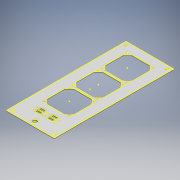
# Autodesk Inventor part: top_panel2
Saved by Autodesk Inventor 2018 (Build 220112000, 112)
## iProperties
Created: 2021-05-16
Part Number: top_panel2
Material: Generic
Document SubType Name: Modeling
Designer: gisen
Density: 1 g/cm^3
Appearance: Default
Author: gisen
Autodesk Inventor part; units mm, degrees
ref_plane "YZ Plane" through (0, 0, 0) normal (1, 0, 0) x (0, 1, 0)
ref_plane "XZ Plane" through (0, 0, 0) normal (0, 1, 0) x (-1, 0, 0)
ref_plane "XY Plane" through (0, 0, 0) normal (0, 0, 1) x (1, 0, 0)
sketch "Sketch1" plane through (0, 0, 0) normal (0, 0, 1) x (1, 0, 0)
  line L0 (-78, 195) -> (78, 195)
  line L1 (78, 195) -> (78, -195)
  line L2 (78, -195) -> (-78, -195)
  line L3 (-78, -195) -> (-78, 195)
  line L4 (-78, 195) -> (78, -195) construction
  line L5 (78, 195) -> (-78, -195) construction
  point P0 (0, 0)
  dimension "d1" = 156
  dimension "d2" = 390
  constraints: 12 end point, 2 midpoint, 2 parallel, 1 horizontal, 1 perpendicular
  measures "d1" distance of L0.start L0.end
  measures "d2" distance of L0.end L1.end
extrude "Extrusion1" add sketch "Sketch1" along normal blind 3
sketch "Sketch2" plane through (0, 0, 3) normal (0, 0, 1) x (1, 0, 0)
  line L0 (-78, -195) -> (78, -195) projected
  line L1 (-78, 195) -> (-78, -195) projected
  arc A0 (-64.4298, -185.2577) -> (-68.2577, -181.4298) centre (-66, -183) ccw
  arc A1 (-69.8472, -183.7153) -> (-66.7153, -186.8472) centre (-68, -185) ccw
  line L2 (-66.7153, -186.8472) -> (-64.4298, -185.2577)
  line L3 (-69.8472, -183.7153) -> (-68.2577, -181.4298)
  line L4 (0, 16.0888) -> (0, -25.3045)
  line L5 (-19.6832, 0) -> (22.709, 0)
  arc A2 (68.2577, -181.4298) -> (64.4298, -185.2577) centre (66, -183) ccw
  arc A3 (66.7153, -186.8472) -> (69.8472, -183.7153) centre (68, -185) ccw
  line L6 (66.7153, -186.8472) -> (64.4298, -185.2577)
  line L7 (69.8472, -183.7153) -> (68.2577, -181.4298)
  arc A4 (-68.2577, 181.4298) -> (-64.4298, 185.2577) centre (-66, 183) ccw
  arc A5 (-66.7153, 186.8472) -> (-69.8472, 183.7153) centre (-68, 185) ccw
  line L8 (-66.7153, 186.8472) -> (-64.4298, 185.2577)
  line L9 (-69.8472, 183.7153) -> (-68.2577, 181.4298)
  arc A6 (64.4298, 185.2577) -> (68.2577, 181.4298) centre (66, 183) ccw
  arc A7 (69.8472, 183.7153) -> (66.7153, 186.8472) centre (68, 185) ccw
  line L10 (66.7153, 186.8472) -> (64.4298, 185.2577)
  line L11 (69.8472, 183.7153) -> (68.2577, 181.4298)
  point P0 (0, 0)
  dimension "d11" = 12
  dimension "d12" = 10
  dimension "d13" = 12
  dimension "d14" = 10
  dimension "d15" = 5.5
  dimension "d16" = 4.5
  constraints: 24 symmetric about line, 20 end point, 16 point on circle, 8 centre point, 8 coincident, 4 tangent, 1 horizontal, 1 vertical, 6 other
  measures "d11" distance from line of L0 point (-66, -183)
  measures "d12" distance from line of L0 point (-68, -185)
  measures "d13" distance from line of L1 point (-66, -183)
  measures "d14" distance from line of L1 point (-68, -185)
  measures "d15" diameter of A0
  measures "d16" diameter of A1
extrude "Extrusion2" cut sketch "Sketch2" against normal up to surface (3 mm away)
sketch "Sketch3" plane through (0, 0, 3) normal (0, 0, 1) x (1, 0, 0)
  line L0 (78, 195) -> (-78, 195) projected
  line L1 (28.4765, 166.7) -> (-28.4765, 166.7)
  circle A0 centre (-41.25, 163.25) radius 2.25
  line L2 (-28.4765, 77.3) -> (28.4765, 77.3)
  circle A1 centre (-41.25, 80.75) radius 2.25
  circle A2 centre (41.25, 80.75) radius 2.25
  circle A3 centre (41.25, 163.25) radius 2.25
  line L3 (44.7, 93.5235) -> (44.7, 150.4765)
  line L4 (-44.7, 150.4765) -> (-44.7, 93.5235)
  arc A4 (28.4765, 77.3) -> (44.7, 93.5235) centre (0, 122) ccw
  arc A5 (44.7, 150.4765) -> (28.4765, 166.7) centre (0, 122) ccw
  arc A6 (-28.4765, 166.7) -> (-44.7, 150.4765) centre (0, 122) ccw
  arc A7 (-44.7, 93.5235) -> (-28.4765, 77.3) centre (0, 122) ccw
  line L5 (28.4765, -17.7) -> (-28.4765, -17.7)
  circle A8 centre (-41.25, -14.25) radius 2.25
  line L6 (-28.4765, 71.7) -> (28.4765, 71.7)
  circle A9 centre (-41.25, 68.25) radius 2.25
  circle A10 centre (41.25, 68.25) radius 2.25
  circle A11 centre (41.25, -14.25) radius 2.25
  line L7 (44.7, 55.4765) -> (44.7, -1.4765)
  line L8 (-44.7, -1.4765) -> (-44.7, 55.4765)
  arc A12 (44.7, 55.4765) -> (28.4765, 71.7) centre (0, 27) ccw
  arc A13 (28.4765, -17.7) -> (44.7, -1.4765) centre (0, 27) ccw
  arc A14 (-44.7, -1.4765) -> (-28.4765, -17.7) centre (0, 27) ccw
  arc A15 (-28.4765, 71.7) -> (-44.7, 55.4765) centre (0, 27) ccw
  circle A16 centre (41.25, -109.25) radius 2.25
  arc A17 (28.4765, -112.7) -> (44.7, -96.4765) centre (0, -68) ccw
  line L9 (44.7, -96.4765) -> (44.7, -39.5235)
  line L10 (-28.4765, -112.7) -> (28.4765, -112.7)
  circle A18 centre (41.25, -26.75) radius 2.25
  arc A19 (44.7, -39.5235) -> (28.4765, -23.3) centre (0, -68) ccw
  circle A20 centre (-41.25, -109.25) radius 2.25
  arc A21 (-44.7, -96.4765) -> (-28.4765, -112.7) centre (0, -68) ccw
  line L11 (-44.7, -39.5235) -> (-44.7, -96.4765)
  line L12 (28.4765, -23.3) -> (-28.4765, -23.3)
  circle A22 centre (-41.25, -26.75) radius 2.25
  arc A23 (-28.4765, -23.3) -> (-44.7, -39.5235) centre (0, -68) ccw
  point P0 (0, 0)
  dimension "d20" = 73
  dimension "d21" = 41.25
  dimension "d22" = 41.25
  dimension "d24" = 44.7
  dimension "d25" = 4.5
  dimension "d27" = 44.7
  dimension "d31" = 360
  constraints: 24 centre point, 24 end point, 24 point on circle, 13 coincident, 2 horizontal, 1 perpendicular, 1 vertical, 13 other
  measures "d20" distance from line of point (0, 122) L0
  measures "d21" horizontal distance of point (0, 122) point (-41.25, 163.25)
  measures "d22" horizontal distance of point (0, 122) point (-41.25, 163.25)
  measures "d24" distance from line of point (0, 122) L1
  measures "d25" diameter of A0
  measures "d27" distance from line of point (0, 122) L2
extrude "Extrusion3" cut sketch "Sketch3" against normal up to surface (3 mm away)
sketch "Sketch4" plane through (0, 0, 3) normal (0, 0, 1) x (1, 0, 0)
  line L0 (-28.5, -131.3505) -> (-11.5, -131.3505)
  line L1 (-11.5, -131.3505) -> (-11.5, -140.3505)
  line L2 (-11.5, -140.3505) -> (-28.5, -140.3505)
  line L3 (-28.5, -140.3505) -> (-28.5, -131.3505)
  line L4 (-28.5, -131.3505) -> (-11.5, -140.3505) construction
  line L5 (-11.5, -131.3505) -> (-28.5, -140.3505) construction
  circle A0 centre (-35, -135.8505) radius 1.65
  circle A1 centre (-5, -135.8505) radius 1.65
  line L6 (0, -126.9429) -> (0, -150.2324)
  line L7 (28.5, -131.3505) -> (11.5, -131.3505)
  line L8 (11.5, -131.3505) -> (11.5, -140.3505)
  line L9 (11.5, -140.3505) -> (28.5, -140.3505)
  line L10 (28.5, -140.3505) -> (28.5, -131.3505)
  line L11 (28.5, -131.3505) -> (11.5, -140.3505) construction
  line L12 (11.5, -131.3505) -> (28.5, -140.3505) construction
  circle A2 centre (35, -135.8505) radius 1.65
  circle A3 centre (5, -135.8505) radius 1.65
  line L13 (-30.7879, -141.8505) -> (-3.35, -141.8505)
  line L14 (-28.5, -152.3505) -> (-11.5, -152.3505)
  line L15 (-11.5, -152.3505) -> (-11.5, -143.3505)
  line L16 (-11.5, -143.3505) -> (-28.5, -143.3505)
  line L17 (-28.5, -143.3505) -> (-28.5, -152.3505)
  line L18 (-28.5, -152.3505) -> (-11.5, -143.3505) construction
  line L19 (-11.5, -152.3505) -> (-28.5, -143.3505) construction
  circle A4 centre (-35, -147.8505) radius 1.65
  circle A5 centre (-5, -147.8505) radius 1.65
  line L20 (28.5, -152.3505) -> (11.5, -152.3505)
  line L21 (11.5, -152.3505) -> (11.5, -143.3505)
  line L22 (11.5, -143.3505) -> (28.5, -143.3505)
  line L23 (28.5, -143.3505) -> (28.5, -152.3505)
  line L24 (28.5, -152.3505) -> (11.5, -143.3505) construction
  line L25 (11.5, -152.3505) -> (28.5, -143.3505) construction
  circle A6 centre (35, -147.8505) radius 1.65
  circle A7 centre (5, -147.8505) radius 1.65
  point P0 (0, 0)
  point P1 (-20, -135.8505)
  point P2 (20, -135.8505)
  point P3 (-20, -147.8505)
  point P4 (20, -147.8505)
  dimension "d37" = 17
  dimension "d38" = 9
  dimension "d39" = 6.5
  dimension "d40" = 4.5
  dimension "d41" = 3.3
  dimension "d42" = 6.5
  dimension "d43" = 4.5
  dimension "d44" = 3.3
  dimension "d45" = 5
  dimension "d46" = 1.5
  constraints: 52 end point, 27 symmetric about line, 8 centre point, 8 coincident, 8 midpoint, 2 horizontal, 2 parallel, 1 perpendicular, 1 vertical, 6 other
  measures "d37" distance of L1.end L2.end
  measures "d38" distance of L0.end L1.end
  measures "d39" distance from line of L3 point (-35, -135.851)
  measures "d40" distance from line of point (-35, -135.851) L0
  measures "d41" diameter of A0
  measures "d42" distance from line of point (-5, -135.851) L1
  measures "d43" distance from line of L0 point (-5, -135.851)
  measures "d44" diameter of A1
  measures "d45" horizontal distance of A1.centre point (0, 0)
  measures "d46" distance between parallel lines of L13 L2
extrude "Extrusion4" cut sketch "Sketch4" against normal up to surface (3 mm away)
sketch "Sketch5" plane through (0, 0, 3) normal (0, 0, 1) x (1, 0, 0)
  line L0 (-78, -195) -> (78, -195) projected
  line L1 (-2.4755, -172.54) -> (2.4755, -172.54)
  line L2 (-2.4755, -187.46) -> (2.4755, -187.46)
  arc A0 (-2.4755, -172.54) -> (-2.4755, -187.46) centre (0, -180) ccw
  arc A1 (2.4755, -187.46) -> (2.4755, -172.54) centre (0, -180) ccw
  point P0 (0, 0)
  dimension "d49" = 15
  dimension "d51" = 7.46
  dimension "d52" = 7.46
  constraints: 4 end point, 4 point on circle, 2 centre point, 2 horizontal, 1 coincident
  measures "d49" distance from line of L0 point (0, -180)
  measures "d51" distance from line of A0.centre L1
  measures "d52" distance from line of point (0, -180) L2
extrude "Extrusion5" cut sketch "Sketch5" against normal up to surface (3 mm away)
sketch "Sketch6" plane through (0, 0, 3) normal (0, 0, 1) x (1, 0, 0)
  line L0 (-2.4755, -172.54) -> (2.4755, -172.54) projected
  arc A0 (2.4755, -187.46) -> (2.4755, -172.54) centre (0, -180) ccw projected
  line L1 (2.4755, -187.46) -> (-2.4755, -187.46) projected
  arc A1 (-2.4755, -172.54) -> (-2.4755, -187.46) centre (0, -180) ccw projected
  line L2 (-11.5, -152.3505) -> (-28.5, -152.3505) projected
  line L3 (-28.5, -152.3505) -> (-28.5, -143.3505) projected
  line L4 (-28.5, -143.3505) -> (-11.5, -143.3505) projected
  line L5 (-11.5, -143.3505) -> (-11.5, -152.3505) projected
  line L6 (11.5, -143.3505) -> (28.5, -143.3505) projected
  line L7 (28.5, -143.3505) -> (28.5, -152.3505) projected
  line L8 (28.5, -152.3505) -> (11.5, -152.3505) projected
  line L9 (11.5, -152.3505) -> (11.5, -143.3505) projected
  line L10 (11.5, -131.3505) -> (28.5, -131.3505) projected
  line L11 (28.5, -131.3505) -> (28.5, -140.3505) projected
  line L12 (28.5, -140.3505) -> (11.5, -140.3505) projected
  line L13 (11.5, -140.3505) -> (11.5, -131.3505) projected
  circle A2 centre (35, -147.8505) radius 1.65 projected
  circle A3 centre (-35, -147.8505) radius 1.65 projected
  circle A4 centre (5, -135.8505) radius 1.65 projected
  circle A5 centre (-5, -135.8505) radius 1.65 projected
  circle A6 centre (-35, -135.8505) radius 1.65 projected
  circle A7 centre (35, -135.8505) radius 1.65 projected
  circle A8 centre (-5, -147.8505) radius 1.65 projected
  circle A9 centre (5, -147.8505) radius 1.65 projected
  line L14 (-11.5, -131.3505) -> (-11.5, -140.3505) projected
  line L15 (-11.5, -140.3505) -> (-28.5, -140.3505) projected
  line L16 (-28.5, -140.3505) -> (-28.5, -131.3505) projected
  line L17 (-28.5, -131.3505) -> (-11.5, -131.3505) projected
  line L18 (28.4765, -17.7) -> (-28.4765, -17.7) projected
  arc A10 (-44.7, -1.4765) -> (-28.4765, -17.7) centre (0, 27) ccw projected
  line L19 (-44.7, -1.4765) -> (-44.7, 55.4765) projected
  arc A11 (-28.4765, 71.7) -> (-44.7, 55.4765) centre (0, 27) ccw projected
  line L20 (-28.4765, 71.7) -> (28.4765, 71.7) projected
  arc A12 (44.7, 55.4765) -> (28.4765, 71.7) centre (0, 27) ccw projected
  line L21 (44.7, 55.4765) -> (44.7, -1.4765) projected
  arc A13 (28.4765, -17.7) -> (44.7, -1.4765) centre (0, 27) ccw projected
  line L22 (-28.4765, -23.3) -> (28.4765, -23.3) projected
  arc A14 (44.7, -39.5235) -> (28.4765, -23.3) centre (0, -68) ccw projected
  line L23 (44.7, -39.5235) -> (44.7, -96.4765) projected
  arc A15 (28.4765, -112.7) -> (44.7, -96.4765) centre (0, -68) ccw projected
  line L24 (28.4765, -112.7) -> (-28.4765, -112.7) projected
  arc A16 (-44.7, -96.4765) -> (-28.4765, -112.7) centre (0, -68) ccw projected
  line L25 (-44.7, -96.4765) -> (-44.7, -39.5235) projected
  arc A17 (-28.4765, -23.3) -> (-44.7, -39.5235) centre (0, -68) ccw projected
  arc A18 (28.4765, 77.3) -> (44.7, 93.5235) centre (0, 122) ccw projected
  line L26 (28.4765, 77.3) -> (-28.4765, 77.3) projected
  arc A19 (-44.7, 93.5235) -> (-28.4765, 77.3) centre (0, 122) ccw projected
  line L27 (-44.7, 93.5235) -> (-44.7, 150.4765) projected
  arc A20 (-28.4765, 166.7) -> (-44.7, 150.4765) centre (0, 122) ccw projected
  line L28 (-28.4765, 166.7) -> (28.4765, 166.7) projected
  arc A21 (44.7, 150.4765) -> (28.4765, 166.7) centre (0, 122) ccw projected
  line L29 (44.7, 150.4765) -> (44.7, 93.5235) projected
  circle A22 centre (-41.25, -26.75) radius 2.25 projected
  circle A23 centre (41.25, -109.25) radius 2.25 projected
  circle A24 centre (-41.25, 68.25) radius 2.25 projected
  circle A25 centre (41.25, 68.25) radius 2.25 projected
  circle A26 centre (41.25, 80.75) radius 2.25 projected
  circle A27 centre (-41.25, 163.25) radius 2.25 projected
  circle A28 centre (-41.25, 80.75) radius 2.25 projected
  circle A29 centre (41.25, 163.25) radius 2.25 projected
  circle A30 centre (41.25, -14.25) radius 2.25 projected
  circle A31 centre (-41.25, -14.25) radius 2.25 projected
  circle A32 centre (41.25, -26.75) radius 2.25 projected
  circle A33 centre (-41.25, -109.25) radius 2.25 projected
  line L30 (-66.7153, 186.8472) -> (-64.4298, 185.2577) projected
  arc A34 (-68.2577, 181.4298) -> (-64.4298, 185.2577) centre (-66, 183) ccw projected
  line L31 (-68.2577, 181.4298) -> (-69.8472, 183.7153) projected
  arc A35 (-66.7153, 186.8472) -> (-69.8472, 183.7153) centre (-68, 185) ccw projected
  arc A36 (69.8472, 183.7153) -> (66.7153, 186.8472) centre (68, 185) ccw projected
  line L32 (69.8472, 183.7153) -> (68.2577, 181.4298) projected
  arc A37 (64.4298, 185.2577) -> (68.2577, 181.4298) centre (66, 183) ccw projected
  line L33 (64.4298, 185.2577) -> (66.7153, 186.8472) projected
  line L34 (66.7153, -186.8472) -> (64.4298, -185.2577) projected
  arc A38 (68.2577, -181.4298) -> (64.4298, -185.2577) centre (66, -183) ccw projected
  line L35 (68.2577, -181.4298) -> (69.8472, -183.7153) projected
  arc A39 (66.7153, -186.8472) -> (69.8472, -183.7153) centre (68, -185) ccw projected
  arc A40 (-69.8472, -183.7153) -> (-66.7153, -186.8472) centre (-68, -185) ccw projected
  line L36 (-69.8472, -183.7153) -> (-68.2577, -181.4298) projected
  arc A41 (-64.4298, -185.2577) -> (-68.2577, -181.4298) centre (-66, -183) ccw projected
  line L37 (-64.4298, -185.2577) -> (-66.7153, -186.8472) projected
  line L38 (78, 195) -> (-78, 195) projected
  line L39 (-78, 195) -> (-78, -195) projected
  line L40 (-78, -195) -> (78, -195) projected
  line L41 (78, -195) -> (78, 195) projected
  point P0 (0, 0)
equation "\"d13\" = d11"
equation "\"d14\" = d12"
equation "\"d27\" = d24"
equation "\"d42\" = d39"
equation "\"d44\" = d41"
equation "\"d26\" = d24"
equation "\"d28\" = d26"
body "Solid1"
